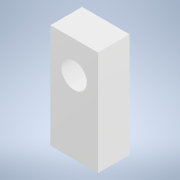
# Autodesk Inventor part: long back plate spacer
Saved by Autodesk Inventor 2022 (Build 260153000, 153)
## iProperties
Created: 2021-05-28
Part Number: long back plate spacer
Material: ABS Plastic
Document SubType Name: Modeling
Designer: benka
Density: 1.06 g/cm^3
Appearance: Smooth - White
Author: benka
Autodesk Inventor part; units mm, degrees
ref_plane "YZ Plane" through (0, 0, 0) normal (1, 0, 0) x (0, 1, 0)
ref_plane "XZ Plane" through (0, 0, 0) normal (0, 1, 0) x (-1, 0, 0)
ref_plane "XY Plane" through (0, 0, 0) normal (0, 0, 1) x (1, 0, 0)
sketch "Sketch1" plane through (0, 0, 0) normal (0, 0, 1) x (1, 0, 0)
  line L0 (7.4982, 17) -> (-0.0018, 17)
  line L1 (-0.0018, 17) -> (-0.0018, 0.5)
  line L2 (7.4982, 17) -> (7.4982, 0.5)
  line L3 (-0.0018, 0.5) -> (7.4982, 0.5)
  circle A0 centre (3.7482, 12) radius 2
  dimension "d5" = 16.5
  dimension "d10" = 4
  dimension "d11" = 5
  dimension "d12" = 7.5
  constraints: 8 end point, 2 parallel, 1 centre point, 1 other
  measures "d5" distance of L0.start L2.end
  measures "d10" diameter of A0
  measures "d11" distance from line of L0 A0.centre
  measures "d12" distance between parallel lines of L2 L1
extrude "Extrusion1" add sketch "Sketch1" along normal blind 5
body "Solid1"
